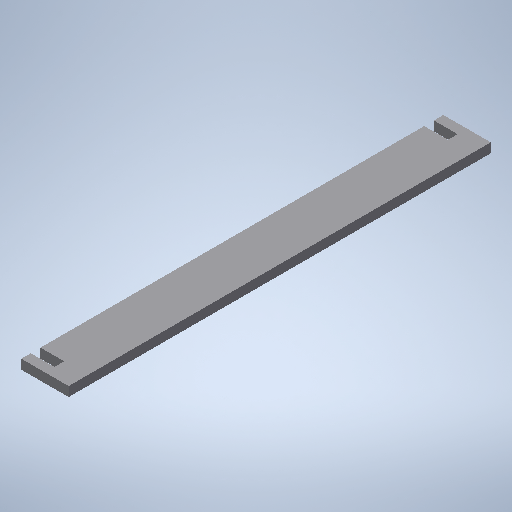
# Autodesk Inventor part: Seguro inf 1
Saved by Autodesk Inventor 2025 (Build 290162000, 162)
## iProperties
Created: 2024-10-28
Part Number: Seguro inf 1
Material: Generic
Document SubType Name: Modeling
Designer: feder
Density: 1 g/cm^3
Appearance: Default
Author: feder
Autodesk Inventor part; units mm, degrees
ref_plane "YZ Plane" through (0, 0, 0) normal (1, 0, 0) x (0, 1, 0)
ref_plane "XZ Plane" through (0, 0, 0) normal (0, 1, 0) x (-1, 0, 0)
ref_plane "XY Plane" through (0, 0, 0) normal (0, 0, 1) x (1, 0, 0)
sketch "Sketch2" plane through (0, 0, 0) normal (0, 1, 0) x (-1, 0, 0)
  line L0 (5.5605, 164.1332) -> (-14.4395, 164.1332)
  line L1 (-14.4395, 164.1332) -> (-14.4395, -14.0668)
  line L2 (-14.4395, -14.0668) -> (5.5605, -14.0668)
  line L3 (5.5605, -14.0668) -> (5.5605, 164.1332)
  line L4 (5.5605, -10.0668) -> (-4.4395, -10.0668)
  line L5 (-4.4395, -10.0668) -> (-4.4395, -5.9668)
  line L6 (-4.4395, -5.9668) -> (5.5605, -5.9668)
  line L7 (5.5605, -5.9668) -> (5.5605, -10.0668)
  line L8 (5.5605, 160.1332) -> (-4.4395, 160.1332)
  line L9 (-4.4395, 160.1332) -> (-4.4395, 156.0332)
  line L10 (-4.4395, 156.0332) -> (5.5605, 156.0332)
  line L11 (5.5605, 156.0332) -> (5.5605, 160.1332)
  point P0 (0, 0)
  point P1 (5.5605, -5.9668)
  dimension "d8" = 178.2
  dimension "d9" = 20
  dimension "d10" = 4.1
  dimension "d11" = 4
  dimension "d12" = 10
  dimension "d15" = 4.1
  dimension "d16" = 4
  dimension "d17" = 10
  constraints: 24 end point, 6 parallel, 3 horizontal, 3 perpendicular, 2 point on line
  measures "d8" distance of L2.end L0.start
  measures "d9" distance of L1.end L2.end
  measures "d10" distance between parallel lines of L6 L4
  measures "d11" distance between parallel lines of L2 L4
  measures "d12" distance between parallel lines of L3 L5
  measures "d15" distance of L8.end L9.end
  measures "d16" distance between parallel lines of L0 L8
  measures "d17" distance of L9.end L10.end
extrude "Extrusion2" add sketch "Sketch2" along normal blind 4 contours L3 L8 L9 L10 L6 L5 L4 L2 L1 L0
body "Solid2"
